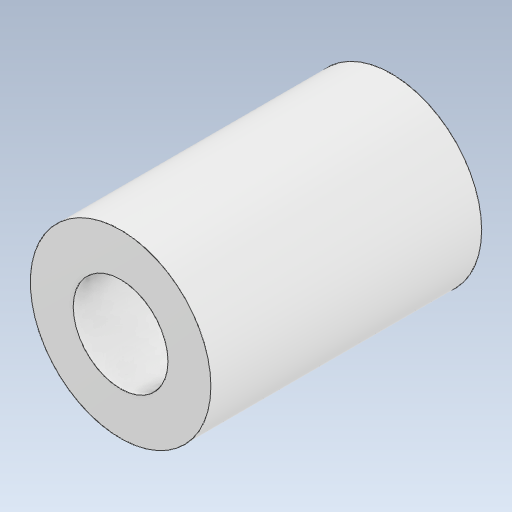
# Autodesk Inventor part: C-2006-4
Saved by Autodesk Inventor 2020 (Build 240168000, 168)
## iProperties
Part Number: C-2006-4
Material: アセタール樹脂、白
Document SubType Name: Modeling
Designer: Masato Kubotera
Density: 1.425 g/cm^3
Appearance: 滑らか - 白
Catalog Web Link: https://www.hirosugi-net.co.jp/shop/g/g5920/
Description: ReadyMade
Author: Masato Kubotera
Autodesk Inventor part; units mm, degrees
ref_plane "YZ Plane" through (0, 0, 0) normal (1, 0, 0) x (0, 1, 0)
ref_plane "XZ Plane" through (0, 0, 0) normal (0, 1, 0) x (-1, 0, 0)
ref_plane "XY Plane" through (0, 0, 0) normal (0, 0, 1) x (1, 0, 0)
sketch "スケッチ1" plane through (0, 0, 0) normal (0, 1, 0) x (-1, 0, 0)
  line L0 (-1.05, 0) -> (-1.05, 6)
  line L1 (-1.05, 6) -> (-2, 6)
  line L2 (-2, 6) -> (-2, 0)
  line L3 (-2, 0) -> (-1.05, 0)
  line L4 (0, 0) -> (0, 6) construction
  dimension "d0" = 6
  dimension "d1" = 2.1
  dimension "d2" = 4
  constraints: 10 end point, 4 perpendicular, 2 point on line, 1 vertical
  measures "d0" distance of L1.end L2.end
  measures "d1" diameter of L0 L4
  measures "d2" diameter of L2 L4
revolve "回転1" add sketch "スケッチ1" angle 360 about axis through (0, 0, 0) along (0, 0, 1)
